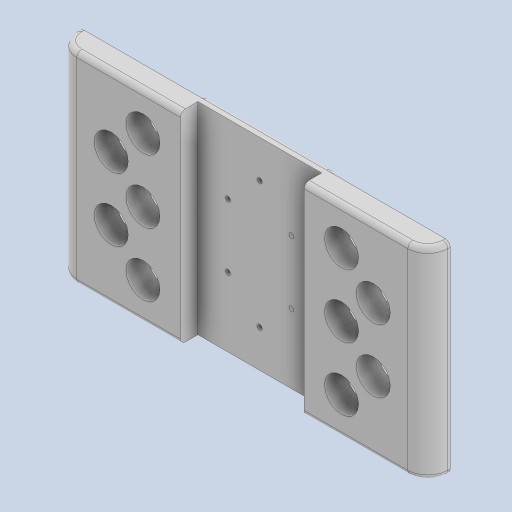
# Autodesk Inventor part: Tabletop Roller Adapter
Saved by Autodesk Inventor 2024 (Build 280153000, 153)
## iProperties
Created: 2025-06-03
Part Number: Tabletop Roller Adapter
Material: Generic
Document SubType Name: Modeling
Designer: Kemper Room 121
Density: 1 g/cm^3
Appearance: Default
Author: Kemper Room 121
Autodesk Inventor part; units mm, degrees
ref_plane "YZ Plane" through (0, 0, 0) normal (1, 0, 0) x (0, 1, 0)
ref_plane "XZ Plane" through (0, 0, 0) normal (0, 1, 0) x (-1, 0, 0)
ref_plane "XY Plane" through (0, 0, 0) normal (0, 0, 1) x (1, 0, 0)
sketch "Sketch1" plane through (0, 0, 0) normal (0, 0, 1) x (1, 0, 0)
  line L0 (0, 0) -> (49.5, 0)
  line L1 (49.5, 0) -> (49.5, 100)
  line L2 (49.5, 100) -> (0, 100)
  line L3 (0, 100) -> (0, 0)
  line L4 (-49.5036, 80.8) -> (99.0036, 80.8)
  line L5 (99.0036, 80.8) -> (99.0036, 0)
  line L6 (99.0036, 0) -> (-49.5036, 0)
  line L7 (-49.5036, 0) -> (-49.5036, 80.8)
  circle A0 centre (64.5, 65.8) radius 6.8036
  circle A1 centre (77.2, 53.1) radius 6.8036
  circle A2 centre (64.5, 40.4) radius 6.8036
  circle A3 centre (64.5, 15) radius 6.8036
  circle A4 centre (77.2, 27.7) radius 6.8036
  line L8 (24.75, -25.8484) -> (24.75, 97.8616)
  circle A5 centre (-15, 65.8) radius 6.8036
  circle A6 centre (-27.7, 53.1) radius 6.8036
  circle A7 centre (-15, 40.4) radius 6.8036
  circle A8 centre (-15, 15) radius 6.8036
  circle A9 centre (-27.7, 27.7) radius 6.8036
  point P0 (24.75, 0)
  point P1 (24.75, 0)
  point P2 (99.0036, 40.4)
  dimension "d0" = 49.5
  dimension "d1" = 100
  dimension "d2" = 0
  dimension "d3" = 13.6071
  dimension "d4" = 13.6071
  dimension "d5" = 15
  dimension "d6" = 12.7
  dimension "d7" = 12.7
  dimension "d8" = 13.6071
  dimension "d9" = 0
  dimension "d10" = 12.7
  dimension "d14" = 25.4
  dimension "d20" = 0
  dimension "d21" = 15
  dimension "d22" = 15
  dimension "d23" = 80.8
  dimension "d24" = 21.8036
  dimension "d25" = 0
  constraints: 18 end point, 10 centre point, 5 symmetric about line, 4 parallel, 3 midpoint, 2 horizontal, 2 perpendicular, 2 vertical, 9 other
  measures "d0" distance of L0.start L0.end
  measures "d1" distance of L0.end L1.end
  measures "d2" distance of point (24.75, 0) point (24.75, 0)
  measures "d3" diameter of A0
  measures "d4" diameter of A1
  measures "d5" distance from line of L1 A0.centre
  measures "d6" horizontal distance of A0.centre A1.centre
  measures "d7" horizontal distance of A0.centre A1.centre
  measures "d8" diameter of A2
  measures "d9" horizontal distance of A0.centre A2.centre
  measures "d10" horizontal distance of A1.centre A2.centre
  measures "d14" distance of A2.centre A3.centre
  measures "d20" distance between parallel lines of L0 L6
  measures "d21" distance from line of L6 A3.centre
  measures "d22" distance from line of L4 A0.centre
  measures "d23" distance of L4.end L5.end
  measures "d24" distance from line of L5 A1.centre
  measures "d25" horizontal distance of point (24.75, 0) L8.start
extrude "Extrusion1" add sketch "Sketch1" along normal blind 2 contours L3 L4 L8 L0 | L6 L7 L4 L3 | L8 L4 L1 L0 | L1 L4 L5 L6
sketch "Sketch2" plane through (0, 0, 2) normal (0, 0, 1) x (1, 0, 0)
  line L0 (-49.5036, 0) -> (99.0036, 0) projected
  line L1 (99.0036, 0) -> (99.0036, 80.8) projected
  line L2 (99.0036, 80.8) -> (-49.5036, 80.8) projected
  line L3 (-49.5036, 80.8) -> (-49.5036, 0) projected
  circle A0 centre (77.2, 27.7) radius 6.8036 projected
  circle A1 centre (64.5, 15) radius 6.8036 projected
  circle A2 centre (64.5, 40.4) radius 6.8036 projected
  circle A3 centre (77.2, 53.1) radius 6.8036 projected
  circle A4 centre (64.5, 65.8) radius 6.8036 projected
  circle A5 centre (-15, 15) radius 6.8036 projected
  circle A6 centre (-27.7, 27.7) radius 6.8036 projected
  circle A7 centre (-15, 40.4) radius 6.8036 projected
  circle A8 centre (-27.7, 53.1) radius 6.8036 projected
  circle A9 centre (-15, 65.8) radius 6.8036 projected
  line L4 (0, 0) -> (49.5, 0)
  line L5 (49.5, 0) -> (49.5, 80.8)
  line L6 (49.5, 80.8) -> (0, 80.8)
  line L7 (0, 80.8) -> (0, 0)
  line L8 (-49.5036, 80.8) -> (99.0036, 80.8)
  line L9 (99.0036, 80.8) -> (99.0036, 0)
  line L10 (99.0036, 0) -> (-49.5036, 0)
  line L11 (-49.5036, 0) -> (-49.5036, 80.8)
  circle A10 centre (-15, 65.8) radius 6.8036
  circle A11 centre (-27.7, 53.1) radius 6.8036
  circle A12 centre (-15, 40.4) radius 6.8036
  circle A13 centre (-27.7, 27.7) radius 6.8036
  circle A14 centre (-15, 15) radius 6.8036
  circle A15 centre (64.5, 40.4) radius 6.8036
  circle A16 centre (77.2, 27.7) radius 6.8036
  circle A17 centre (64.5, 15) radius 6.8036
  circle A18 centre (77.2, 53.1) radius 7.25
  circle A19 centre (64.5, 65.8) radius 6.8036
  dimension "d28" = 49.5
  dimension "d29" = 15
  dimension "d30" = 15
  constraints: 16 end point, 10 centre point, 10 coincident, 9 concentric, 4 parallel, 2 horizontal, 2 perpendicular, 1 point on line
  measures "d28" distance between parallel lines of L7 L5
  measures "d29" distance from line of A2.centre L5
  measures "d30" distance from line of L7 A7.centre
extrude "Extrusion2" add sketch "Sketch2" along normal blind 7 contours L3 L2 L7 L0 | L5 L2 L1 L0 | A18
sketch "Sketch3" plane through (0, 0, 2) normal (0, 0, 1) x (1, 0, 0)
  line L0 (49.5, 0) -> (49.5, 80.8) projected
  line L1 (49.5, 80.8) -> (0, 80.8) projected
  line L2 (0, 80.8) -> (0, 0) projected
  line L3 (0, 0) -> (49.5, 0) projected
  circle A0 centre (24.75, 65.8) radius 1
  circle A1 centre (12.05, 53.1) radius 1
  circle A2 centre (37.45, 53.1) radius 1
  line L4 (-69.5115, 40.4) -> (155.6489, 40.4)
  circle A3 centre (24.75, 15) radius 1
  circle A4 centre (12.05, 27.7) radius 1
  circle A5 centre (37.45, 27.7) radius 1
  point P0 (24.75, 80.8)
  dimension "d33" = 2
  dimension "d34" = 2
  dimension "d35" = 0
  dimension "d36" = 12.7
  dimension "d37" = 12.7
  dimension "d38" = 15
  dimension "d39" = 2
  dimension "d40" = 0
  dimension "d41" = 12.7
  dimension "d42" = 12.7
  constraints: 6 centre point, 3 symmetric about line, 2 end point, 1 horizontal, 1 midpoint, 3 other
  measures "d33" diameter of A0
  measures "d34" diameter of A1
  measures "d35" horizontal distance of point (24.75, 80.8) A0.centre
  measures "d36" horizontal distance of A0.centre A1.centre
  measures "d37" horizontal distance of A0.centre A1.centre
  measures "d38" distance from line of L1 A0.centre
  measures "d39" diameter of A2
  measures "d40" vertical distance of A1.centre A2.centre
  measures "d41" horizontal distance of A0.centre A2.centre
  measures "d42" distance from line of A1.centre L4
extrude "Extrusion3" cut sketch "Sketch3" against normal through all contours A0 | A1 | A2 | A3 | A4 | A5
sketch "Sketch4" plane through (0, 0, 0) normal (0, 0, -1) x (-1, 0, 0)
  circle A0 centre (-37.45, 53.1) radius 1 projected
  circle A1 centre (-24.75, 15) radius 1 projected
  circle A2 centre (-24.75, 65.8) radius 1 projected
  circle A3 centre (-12.05, 27.7) radius 1 projected
  circle A4 centre (-37.45, 27.7) radius 1 projected
  circle A5 centre (-12.05, 53.1) radius 1 projected
  line L0 (-49.5, 0) -> (-49.5, 80.8) projected
  line L1 (-49.5, 80.8) -> (0, 80.8) projected
  line L2 (0, 80.8) -> (0, 0) projected
  line L3 (0, 0) -> (-49.5, 0) projected
  line L4 (0, 80.8) -> (49.5036, 80.8) projected
  line L5 (49.5036, 80.8) -> (49.5036, 0) projected
  line L6 (49.5036, 0) -> (0, 0) projected
  line L7 (0, 0) -> (0, 80.8) projected
  circle A6 centre (27.7, 53.1) radius 6.8036 projected
  circle A7 centre (15, 15) radius 6.8036 projected
  circle A8 centre (27.7, 27.7) radius 6.8036 projected
  circle A9 centre (15, 40.4) radius 6.8036 projected
  circle A10 centre (15, 65.8) radius 6.8036 projected
  line L8 (-49.5, 0) -> (-99.0036, 0) projected
  line L9 (-99.0036, 0) -> (-99.0036, 80.8) projected
  line L10 (-99.0036, 80.8) -> (-49.5, 80.8) projected
  line L11 (-49.5, 80.8) -> (-49.5, 0) projected
  circle A11 centre (-64.5, 65.8) radius 6.8036 projected
  circle A12 centre (-77.2, 53.1) radius 6.8036 projected
  circle A13 centre (-64.5, 40.4) radius 6.8036 projected
  circle A14 centre (-64.5, 15) radius 6.8036 projected
  circle A15 centre (-77.2, 27.7) radius 6.8036 projected
  line L12 (-49.5, 56.85) -> (0, 56.85)
  line L13 (0, 56.85) -> (0, 61.85)
  line L14 (0, 61.85) -> (-49.5, 61.85)
  line L15 (-49.5, 61.85) -> (-49.5, 56.85)
  line L16 (-49.5, 37.9) -> (0, 37.9)
  line L17 (0, 37.9) -> (0, 42.9)
  line L18 (0, 42.9) -> (-49.5, 42.9)
  line L19 (-49.5, 42.9) -> (-49.5, 37.9)
  line L20 (-49.5, 0) -> (-49.5, 80.8) projected
  line L21 (-49.5, 18.95) -> (0, 18.95)
  line L22 (0, 18.95) -> (0, 23.95)
  line L23 (0, 23.95) -> (-49.5, 23.95)
  line L24 (-49.5, 23.95) -> (-49.5, 18.95)
  line L25 (-49.5, 0) -> (0, 0)
  line L26 (0, 0) -> (0, 5)
  line L27 (0, 5) -> (-49.5, 5)
  line L28 (-49.5, 5) -> (-49.5, 0)
  line L29 (-49.5, 80.8) -> (0, 80.8)
  line L30 (0, 80.8) -> (0, 75.8)
  line L31 (0, 75.8) -> (-49.5, 75.8)
  line L32 (-49.5, 75.8) -> (-49.5, 80.8)
  circle A16 centre (0, 40.4) radius 2.5
  line L33 (0, 80.8) -> (0, 0) projected
  circle A17 centre (0, 59.35) radius 2.5
  circle A18 centre (0, 78.3) radius 2.5
  circle A19 centre (-49.5, 78.3) radius 2.5
  circle A20 centre (-49.5, 59.35) radius 2.5
  circle A21 centre (-49.5, 40.4) radius 2.5
  circle A22 centre (-49.5, 21.45) radius 2.5
  circle A23 centre (0, 21.45) radius 2.5
  circle A24 centre (0, 2.5) radius 2.5
  circle A25 centre (-49.5, 2.5) radius 2.5
  point P0 (0, 18.95)
  point P1 (0, 37.9)
  point P2 (0, 56.85)
  dimension "d45" = 5
  dimension "d46" = 5
  dimension "d47" = 5
  dimension "d48" = 5
  dimension "d49" = 5
  dimension "d50" = 0
  dimension "d51" = 37.9
  dimension "d52" = 18.95
  dimension "d53" = 18.95
  constraints: 40 end point, 10 midpoint, 10 parallel, 7 point on line, 5 coincident, 5 horizontal, 5 perpendicular, 35 other
  measures "d45" distance between parallel lines of L1 L31
  measures "d46" distance between parallel lines of L14 L12
  measures "d47" distance between parallel lines of L18 L16
  measures "d48" distance between parallel lines of L23 L21
  measures "d49" distance between parallel lines of L27 L3
  measures "d50" distance of point (-49.5, 40.4) point (-49.5, 40.4)
  measures "d51" distance of point (-49.5, 2.5) point (-49.5, 40.4)
  measures "d52" distance of point (-49.5, 2.5) point (-49.5, 21.45)
  measures "d53" distance of point (-49.5, 78.3) point (-49.5, 59.35)
extrude "Extrusion4" add sketch "Sketch4" along normal blind 2 contours A25 L0 | A25 L27 A24 L3 | L0 A25 | A24 L2 | L2 A24 | A22 L0 | A22 L23 A23 L21 | L0 A22 | A23 L2 | L2 A23 | A19 L0 | L1 A18 L31 A19 | L0 A19 | A21 L0 | A21 L18 A16 L16 | L0 A21 | A18 L2 | L2 A18 | A16 L2 | L2 A16 | A20 L0 | L14 A17 L12 A20 | L0 A20 | A17 L2 | L2 A17
fillet "Fillet1" radius 2 20 edges at (24.75, 0, -2) (-2.5, 2.5, -2) (24.75, 5, -2) (52, 2.5, -2) (-2.5, 21.45, -2) (24.75, 23.95, -2) (52, 21.45, -2) (24.75, 18.95, -2) (-2.5, 40.4, -2) (24.75, 42.9, -2) (52, 40.4, -2) (24.75, 37.9, -2) (-2.5, 59.35, -2) (24.75, 61.85, -2) (52, 59.35, -2) (24.75, 56.85, -2) (-2.5, 78.3, -2) (24.75, 80.8, -2) (52, 78.3, -2) (24.75, 75.8, -2)
fillet "Fillet2" radius 2 8 edges at (-24.7518, 0, 9) (-49.5036, 0, 4.5) (-24.7518, 80.8, 9) (99.0036, 0, 4.5) (74.2518, 0, 9) (74.2518, 80.8, 9) (-49.5036, 80.8, 4.5) (99.0036, 80.8, 4.5)
fillet "Fillet3" radius 8 6 edges at (-48.9178, 0.5858, 8.4142) (-48.9178, 80.2142, 8.4142) (-49.5036, 40.4, 9) (98.4178, 80.2142, 8.4142) (98.4178, 0.5858, 8.4142) (99.0036, 40.4, 9)
equation "\"d4\" = d3"
equation "\"d8\" = d3"
equation "\"d34\" = d33"
equation "\"d39\" = d33"
equation "\"d46\" = d45"
equation "\"d47\" = d46"
equation "\"d48\" = d46"
equation "\"d49\" = d45"
equation "\"d52\" = 0.5 * d51"
equation "\"d53\" = d52"
body "Solid1"
